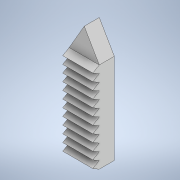
# Autodesk Inventor part: Prensas coletor
Saved by Autodesk Inventor 2021 (Build 250183000, 183)
## iProperties
Created: 2020-09-23
Part Number: Prensas coletor
Material: Genérico
Document SubType Name: Modeling
Designer: rapha
Density: 1 g/cm^3
Appearance: Padrão
Author: rapha
Autodesk Inventor part; units mm, degrees
ref_plane "YZ Plane" through (0, 0, 0) normal (1, 0, 0) x (0, 1, 0)
ref_plane "XZ Plane" through (0, 0, 0) normal (0, 1, 0) x (-1, 0, 0)
ref_plane "XY Plane" through (0, 0, 0) normal (0, 0, 1) x (1, 0, 0)
sketch "Esboço1" plane through (0, 0, 0) normal (0, 0, 1) x (1, 0, 0)
  line L0 (0, 0) -> (0, 30)
  line L1 (10, 0) -> (10, 30)
  line L2 (0, 0) -> (10, 0)
  line L3 (0, 30) -> (5, 38.6603)
  line L4 (5, 38.6603) -> (10, 30)
  dimension "d0" = 30
  dimension "d3" = 30
  dimension "d4" = 10
  constraints: 10 end point, 2 vertical, 1 horizontal
  measures "d0" distance of L0.start L0.end
  measures "d3" distance of L1.start L1.end
  measures "d4" distance of L0.end L3.end
extrude "Extrusão1" add sketch "Esboço1" along normal blind 5
sketch "Esboço3" plane through (10, 0, 0) normal (1, 0, 0) x (0, 0, -1)
  line L0 (-5, 30) -> (-5, 0) projected
  line L1 (-5, 0) -> (-2.5, 0) construction
  line L2 (-5, 0) -> (-7.1651, 1.25)
  line L3 (-5, 0) -> (-2.5, 0) construction
  line L4 (-7.1651, 1.25) -> (-5, 2.5)
  line L5 (-5, 2.5) -> (-7.1651, 3.75)
  line L6 (-7.1651, 3.75) -> (-5, 5)
  line L7 (-5, 5) -> (-7.1651, 6.25)
  line L8 (-7.1651, 6.25) -> (-5, 7.5)
  line L9 (-5, 7.5) -> (-7.1651, 8.75)
  line L10 (-7.1651, 8.75) -> (-5, 10)
  line L11 (-5, 10) -> (-7.1651, 11.25)
  line L12 (-5, 10) -> (-2.5, 10) construction
  line L13 (-7.1651, 11.25) -> (-5, 12.5)
  line L14 (-5, 12.5) -> (-12.5939, 12.5) construction
  line L15 (-5, 25) -> (-7.1651, 23.75)
  line L16 (-7.1651, 23.75) -> (-5, 22.5)
  line L17 (-5, 22.5) -> (-7.1651, 21.25)
  line L18 (-7.1651, 21.25) -> (-5, 20)
  line L19 (-5, 20) -> (-7.1651, 18.75)
  line L20 (-7.1651, 18.75) -> (-5, 17.5)
  line L21 (-5, 17.5) -> (-7.1651, 16.25)
  line L22 (-7.1651, 16.25) -> (-5, 15)
  line L23 (-5, 15) -> (-7.1651, 13.75)
  line L24 (-7.1651, 13.75) -> (-5, 12.5)
  line L25 (-5, 25) -> (-7.1651, 26.25)
  line L26 (-7.1651, 26.25) -> (-5, 27.5)
  line L27 (-5, 27.5) -> (-7.1651, 28.75)
  line L28 (-7.1651, 28.75) -> (-5, 30)
  line L29 (-5, 30) -> (-5, 38.6603) projected
  line L30 (-5, 30) -> (-5, 0)
  point P0 (0, 0)
  dimension "d10" = 2.5
  dimension "d11" = 150
  dimension "d12" = 2.5
  dimension "d13" = 2.5
  dimension "d14" = 2.5
  dimension "d15" = 2.5
  dimension "d16" = 150
  constraints: 58 end point, 10 symmetric about line, 6 point on line, 4 horizontal, 2 equal length, 1 parallel, 1 vertical
  measures "d10" distance of L0.end L2.end
  measures "d11" angle of L3 L2
  measures "d12" distance of L2.end L4.end
  measures "d13" distance of L6.end L7.end
  measures "d14" distance of L8.end L9.end
  measures "d15" distance of L10.end L11.end
  measures "d16" angle of L12 L11
extrude "Extrusão2" add sketch "Esboço3" against normal blind 10
sketch "Esboço4" plane through (0, 0, 0) normal (0, 0, -1) x (-1, 0, 0)
  circle A0 centre (-5, 5) radius 2.5
  point P0 (0, 0)
  dimension "d19" = 5
  constraints: 1 centre point
  measures "d19" diameter of A0
extrude "Extrusão3" add sketch "Esboço4" along normal blind 1
